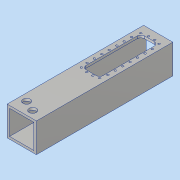
# Autodesk Inventor part: Hull_Alu
Saved by Autodesk Inventor 2018 (Build 220112000, 112)
## iProperties
Created: 2019-08-01
Part Number: Hull_Alu
Material: Aluminum 6061
Document SubType Name: Modeling
Designer: Derek Wider
Density: 2.7 g/cm^3
Appearance: Aluminum - Flat
Author: Derek Wider
Autodesk Inventor part; units mm, degrees
ref_plane "YZ Plane" through (0, 0, 0) normal (1, 0, 0) x (0, 1, 0)
ref_plane "XZ Plane" through (0, 0, 0) normal (0, 1, 0) x (-1, 0, 0)
ref_plane "XY Plane" through (0, 0, 0) normal (0, 0, 1) x (1, 0, 0)
sketch "Sketch1" plane through (0, 0, 0) normal (0, 0, 1) x (1, 0, 0)
  line L0 (0, 0) -> (38.1, 0)
  line L1 (38.1, 0) -> (38.1, 38.1)
  line L2 (38.1, 38.1) -> (0, 38.1)
  line L3 (0, 38.1) -> (0, 0)
  line L4 (3.175, 34.925) -> (34.925, 34.925)
  line L5 (34.925, 34.925) -> (34.925, 3.175)
  line L6 (34.925, 3.175) -> (3.175, 3.175)
  line L7 (3.175, 3.175) -> (3.175, 34.925)
  dimension "d0" = 38.1
  dimension "d1" = 38.1
  dimension "d2" = 3.175
  constraints: 16 end point, 4 parallel, 2 perpendicular, 1 horizontal, 3 other
  measures "d0" distance of L2.end L1.end
  measures "d1" distance of L1.end L0.end
  measures "d2" distance between parallel lines of L2 L4
extrude "Extrusion1" add sketch "Sketch1" along normal blind 177.8
sketch "Sketch2" plane through (0, 38.1, 0) normal (0, 1, 0) x (1, 0, 0)
  line L0 (12.5095, -87.63) -> (25.5905, -87.63)
  line L1 (30.353, -82.8675) -> (30.353, -16.1925)
  line L2 (25.5905, -11.43) -> (12.5095, -11.43)
  line L3 (7.747, -16.1925) -> (7.747, -82.8675)
  line L4 (38.1, 0) -> (0, 0) projected
  arc A0 (7.747, -82.8675) -> (12.5095, -87.63) centre (12.5095, -82.8675) ccw
  arc A1 (25.5905, -87.63) -> (30.353, -82.8675) centre (25.5905, -82.8675) ccw
  arc A2 (30.353, -16.1925) -> (25.5905, -11.43) centre (25.5905, -16.1925) ccw
  arc A3 (12.5095, -11.43) -> (7.747, -16.1925) centre (12.5095, -16.1925) ccw
  point P0 (30.353, -11.43)
  point P1 (30.353, -87.63)
  point P2 (7.747, -11.43)
  point P3 (19.05, -11.43)
  point P4 (19.05, 0)
  dimension "d5" = 22.606
  dimension "d6" = 76.2
  dimension "d7" = 11.43
  dimension "d8" = 4.7625
  constraints: 8 end point, 8 point on circle, 8 tangent, 6 point on line, 4 centre point, 3 equal radius, 2 midpoint, 2 parallel, 1 horizontal, 1 perpendicular, 1 vertical alignment
  measures "d5" distance of point (30.353, -11.43) point (7.747, -11.43)
  measures "d6" distance of point (30.353, -87.63) point (30.353, -11.43)
  measures "d7" distance between parallel lines of L4 L2
  measures "d8" radius of A0
extrude "Extrusion2" cut sketch "Sketch2" against normal blind 3.175
sketch "Sketch3" plane through (0, 38.1, 0) normal (0, 1, 0) x (1, 0, 0)
  circle A0 centre (7.112, -10.795) radius 1.289
  line L0 (0, 0) -> (0, -177.8) projected
  line L1 (12.5095, -11.43) -> (25.5905, -11.43) projected
  line L2 (7.747, -82.8675) -> (7.747, -16.1925) projected
  circle A1 centre (30.988, -10.795) radius 1.289
  circle A2 centre (7.112, -88.265) radius 1.289
  circle A3 centre (30.988, -88.265) radius 1.289
  circle A4 centre (5.461, -21.1137) radius 1.2891
  circle A5 centre (32.639, -21.1137) radius 1.2891
  circle A6 centre (5.461, -30.7975) radius 1.2891
  circle A7 centre (32.639, -30.7975) radius 1.2891
  circle A8 centre (5.461, -40.4812) radius 1.2891
  circle A9 centre (32.639, -40.4812) radius 1.2891
  circle A10 centre (5.461, -50.165) radius 1.2891
  circle A11 centre (32.639, -50.165) radius 1.2891
  circle A12 centre (5.461, -59.8487) radius 1.2891
  circle A13 centre (32.639, -59.8487) radius 1.2891
  circle A14 centre (5.461, -69.5325) radius 1.2891
  circle A15 centre (32.639, -69.5325) radius 1.2891
  circle A16 centre (5.461, -79.2162) radius 1.2891
  circle A17 centre (32.639, -79.2162) radius 1.2891
  circle A18 centre (15.7048, -9.144) radius 1.2891
  circle A19 centre (23.6626, -9.144) radius 1.2891
  circle A20 centre (15.7048, -89.916) radius 1.2891
  circle A21 centre (23.6626, -89.916) radius 1.2891
  dimension "d11" = 2.5781
  dimension "d14" = 0.635
  dimension "d15" = 0.635
  dimension "d18" = 23.876
  dimension "d21" = 77.47
  dimension "d24" = 2.5781
  dimension "d25" = 2.286
  dimension "d26" = 9.6837
  dimension "d29" = 27.178
  dimension "d32" = 9.6837
  dimension "d35" = 2.5781
  dimension "d36" = 7.9578
  dimension "d37" = 2.286
  dimension "d40" = 7.9578
  dimension "d43" = 80.772
  constraints: 22 centre point, 3 horizontal, 3 vertical, 38 other
  measures "d11" diameter of A0
  measures "d14" distance from line of A0.centre L2
  measures "d15" distance from line of A0.centre L1
  measures "d18" distance of A0.centre A1.centre
  measures "d21" distance of A0.centre A2.centre
  measures "d24" diameter of A4
  measures "d25" distance from line of A4.centre L2
  measures "d26" distance from line of A4.centre L1
  measures "d29" distance of A4.centre A5.centre
  measures "d32" distance of A4.centre A6.centre
  measures "d35" diameter of A18
  measures "d36" distance from line of A18.centre L2
  measures "d37" distance from line of A18.centre L1
  measures "d40" distance of A18.centre A19.centre
  measures "d43" distance of A18.centre A20.centre
extrude "Extrusion3" cut sketch "Sketch3" against normal blind 3.175
sketch "Sketch4" plane through (0, 0, 0) normal (0, -1, 0) x (1, 0, 0)
  circle A0 centre (19.05, 82.55) radius 1.2891
  line L0 (0, 0) -> (38.1, 0) projected
  line L1 (38.1, 0) -> (38.1, 177.8) projected
  circle A1 centre (19.05, 95.25) radius 1.2891
  point P0 (19.05, 0)
  dimension "d48" = 2.5781
  dimension "d49" = 82.55
  dimension "d52" = 12.7
  constraints: 2 centre point, 1 midpoint, 1 vertical, 1 vertical alignment, 2 other
  measures "d48" diameter of A0
  measures "d49" distance from line of L0 A0.centre
  measures "d52" distance of A0.centre A1.centre
extrude "Extrusion4" cut sketch "Sketch4" against normal blind 3.175
sketch "Sketch5" plane through (0, 0, 0) normal (0, -1, 0) x (1, 0, 0)
  circle A0 centre (19.05, 114.3) radius 2.3813
  line L0 (0, 0) -> (38.1, 0) projected
  point P0 (19.05, 0)
  dimension "d59" = 4.7625
  dimension "d60" = 114.3
  constraints: 1 centre point, 1 midpoint, 1 vertical alignment
  measures "d59" diameter of A0
  measures "d60" distance from line of L0 A0.centre
extrude "Extrusion5" cut sketch "Sketch5" against normal blind 3.175
sketch "Sketch6" plane through (0, 38.1, 0) normal (0, 1, 0) x (1, 0, 0)
  circle A0 centre (9.525, -161.925) radius 4.7625
  line L0 (38.1, -177.8) -> (0, -177.8) projected
  line L1 (0, 0) -> (0, -177.8) projected
  circle A1 centre (23.8125, -168.275) radius 4.7625
  line L2 (38.1, 0) -> (38.1, -177.8) projected
  dimension "d63" = 15.875
  dimension "d64" = 9.525
  dimension "d65" = 9.525
  dimension "d66" = 9.525
  dimension "d67" = 14.2875
  dimension "d68" = 9.525
  constraints: 2 centre point
  measures "d63" distance from line of A0.centre L0
  measures "d64" distance from line of A0.centre L1
  measures "d65" diameter of A0
  measures "d66" distance from line of L0 A1.centre
  measures "d67" distance from line of L2 A1.centre
  measures "d68" diameter of A1
extrude "Extrusion6" cut sketch "Sketch6" against normal blind 3.175
body "Solid1"
